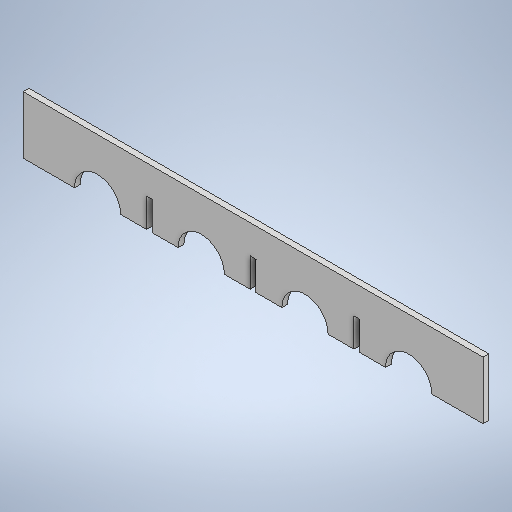
# Autodesk Inventor part: BSH 084 amplifier bottom
Saved by Autodesk Inventor 2025 (Build 290162010, 162A)
## iProperties
Created: 2024-08-04
Part Number: BSH 084 amplifier bottom
Material: Stainless Steel
Document SubType Name: Sheet Metal
Designer: pokla
Density: 8 g/cm^3
Sheet Metal Rule: AISI304 2mm Die16
Appearance: Default
Author: pokla
Autodesk Inventor part; units mm, degrees
ref_plane "YZ Plane" through (0, 0, 0) normal (1, 0, 0) x (0, 1, 0)
ref_plane "XZ Plane" through (0, 0, 0) normal (0, 1, 0) x (-1, 0, 0)
ref_plane "XY Plane" through (0, 0, 0) normal (0, 0, 1) x (1, 0, 0)
sketch "Sketch1" plane through (0, 0, 0) normal (0, 0, 1) x (1, 0, 0)
  circle A0 centre (0, 0) radius 400 construction
  line L0 (-399, 5) -> (399, 5)
  line L1 (399, 5) -> (399, -5)
  line L2 (399, -5) -> (-399, -5)
  line L3 (-399, -5) -> (-399, 5)
  line L4 (-399, 5) -> (399, -5) construction
  dimension "d0" = 800
  dimension "d1" = 10
  dimension "d2" = 798
  constraints: 10 end point, 3 coincident, 2 parallel, 1 centre point, 1 horizontal, 1 midpoint, 1 perpendicular
  measures "d0" diameter of A0
  measures "d1" distance of L0.end L1.end
  measures "d2" distance of L0.start L0.end
extrude "Extrusion1" add sketch "Sketch1" along normal blind 100
sketch "Sketch2" plane through (-399, -5, 0) normal (0, -1, 0) x (1, 0, 0)
  circle A0 centre (309, 0) radius 40
  line L0 (0, 0) -> (798, 0) projected
  circle A1 centre (129, 0) radius 40
  circle A2 centre (489, 0) radius 40
  circle A3 centre (669, 0) radius 40
  line L1 (394, 50) -> (404, 50)
  line L2 (404, 50) -> (404, 0)
  line L3 (404, 0) -> (394, 0)
  line L4 (394, 0) -> (394, 50)
  line L5 (214, 50) -> (224, 50)
  line L6 (224, 50) -> (224, 0)
  line L7 (224, 0) -> (214, 0)
  line L8 (214, 0) -> (214, 50)
  line L9 (574, 50) -> (584, 50)
  line L10 (584, 50) -> (584, 0)
  line L11 (584, 0) -> (574, 0)
  line L12 (574, 0) -> (574, 50)
  point P0 (399, 0)
  point P1 (399, 0)
  point P2 (399, 0)
  point P3 (399, 0)
  point P4 (709, 0)
  point P5 (629, 0)
  point P6 (529, 0)
  point P7 (449, 0)
  point P8 (269, 0)
  point P9 (349, 0)
  point P10 (169, 0)
  point P11 (89, 0)
  point P12 (399, 0)
  point P13 (219, 0)
  point P14 (399, 0)
  point P15 (399, 0)
  point P16 (579, 0)
  point P17 (399, 0)
  point P18 (399, 0)
  point P19 (574, 0)
  point P20 (584, 0)
  point P21 (214, 0)
  point P22 (224, 0)
  dimension "d5" = 80
  dimension "d7" = 90
  dimension "d8" = 80
  dimension "d9" = 180
  dimension "d10" = 80
  dimension "d11" = 80
  dimension "d12" = 90
  dimension "d13" = 180
  dimension "d24" = 10
  dimension "d25" = 50
  dimension "d26" = 10
  dimension "d27" = 50
  dimension "d28" = 180
  dimension "d29" = 10
  dimension "d30" = 50
  dimension "d31" = 180
  constraints: 24 end point, 6 parallel, 4 centre point, 3 horizontal, 3 horizontal alignment, 3 midpoint, 3 perpendicular, 12 other
  measures "d5" diameter of A0
  measures "d7" distance of point (399, 0) A0.centre
  measures "d8" diameter of A1
  measures "d9" distance of A0.centre A1.centre
  measures "d10" diameter of A2
  measures "d11" diameter of A3
  measures "d12" distance of A2.centre point (399, 0)
  measures "d13" distance of A3.centre A2.centre
  measures "d24" distance of L1.start L1.end
  measures "d25" distance of L3.end L1.start
  measures "d26" distance of L5.start L5.end
  measures "d27" distance of L7.end L5.start
  measures "d28" distance of point (399, 0) point (219, 0)
  measures "d29" distance of L9.start L9.end
  measures "d30" distance of L11.end L9.start
  measures "d31" distance of point (579, 0) point (399, 0)
extrude "Extrusion2" cut sketch "Sketch2" against normal through all contours L0 A0 | L0 A1 | L0 L8 L5 L6 | A3 L0 | L12 L9 L10 L0 | A2 L0 | L4 L1 L2 L0 picked at (302.3333, 20.5179) picked at (130.5738, 20.5179) picked at (658.2131, 7.8371) picked at (497.9217, 9.9086)
equation "\"d26\" = d24"
equation "\"d27\" = d25"
equation "\"d29\" = d24"
equation "\"d30\" = d25"
equation "\"BendReliefWidth\" = Thickness"
equation "\"BendReliefDepth\" = 0.5 * Thickness"
equation "\"CornerReliefSize\" = 4 * Thickness"
equation "\"MinimumRemnant\" = 2 * Thickness"
equation "\"TransitionRadius\" = BendRadius"
equation "\"JacobiRadiusSize\" = BendRadius"
equation "\"GapSize\" = Thickness"
equation "\"Thickness\" = 2"
equation "\"BendRadius\" = 2.75"
body "Solid1"
